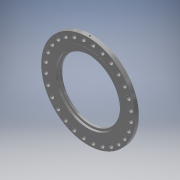
# Autodesk Inventor part: A1-19010-200-01 30in CL300 RFBL flange - thinned
Saved by Autodesk Inventor 2017.3 (Build 213257000, 257)
## iProperties
Created: 2014-07-18
Part Number: A1-19010-200-01 30in CL300 RFBL flange - thinned
Material: Steel, Mild
Document SubType Name: Modeling
Designer: Graeme_Van_Dongen
Density: 7.86 g/cm^3
Appearance: Steel
Mass: 182237 g
Surface Area: 14853.8 cm^2
Volume: 23185.3 cm^3
Description: Ø30" CLASS 300 RFBL FLANGE, A516 Gr.70N, ASME B16.47 Ser.A, 50mm THICK
Author: Graeme_Van_Dongen
Autodesk Inventor part; units mm, degrees
ref_plane "YZ Plane" through (0, 0, 0) normal (1, 0, 0) x (0, 1, 0)
ref_plane "XY Plane" through (0, 0, 0) normal (0, 0, 1) x (1, 0, 0)
sketch "Sketch1" plane through (0, 0, 0) normal (0, 0, 1) x (1, 0, 0)
  circle A0 centre (0, 0) radius 546.1
  dimension "d0" = 1092.2
  constraints: 1 centre point, 1 coincident
  measures "d0" diameter of A0
extrude "Extrusion1" add sketch "Sketch1" along normal blind 48.4125
sketch "Sketch2" plane through (0, 0, 48.4125) normal (0, 0, 1) x (1, 0, 0)
  circle A0 centre (0, 0) radius 428.625
  dimension "d3" = 857.25
  constraints: 1 centre point, 1 coincident
  measures "d3" diameter of A0
extrude "Extrusion2" add sketch "Sketch2" along normal blind 1.5875
sketch "Sketch3" plane through (0, 0, 50) normal (0, 0, 1) x (1, 0, 0)
  circle A0 centre (0, 0) radius 374.65
  dimension "d6" = 749.3
  dimension "d32" = 0
  constraints: 1 centre point, 1 coincident
  measures "d6" diameter of A0
  measures "d32" distance of point (0, 0) A0.centre
extrude "Extrusion3" cut sketch "Sketch3" against normal blind 25.4
sketch "Sketch4" plane through (0, 0, 50) normal (0, 0, 1) x (1, 0, 0)
  circle A0 centre (0, 0) radius 349.25
  circle A1 centre (0, 0) radius 374.65 construction
  dimension "d9" = 698.5
  constraints: 1 centre point, 1 concentric
  measures "d9" diameter of A0
extrude "Extrusion4" cut sketch "Sketch4" against normal through all
sketch "Sketch5" plane through (0, 0, 50) normal (0, 0, 1) x (1, 0, 0)
  line L0 (-495.3407, -55.8115) -> (495.3407, 55.8115)
  line L1 (-495.3407, -55.8115) -> (501.6093, -55.8115) construction
  point P0 (0, 0)
  point P1 (0, 0)
  dimension "d12" = 996.95
  dimension "d13" = 6.429
  constraints: 4 end point, 2 coincident, 1 equal length, 1 horizontal, 1 midpoint
  measures "d12" distance of L0.start L0.end
  measures "d13" angle of L1 L0
hole "Hole1" at (495.3407, 55.8115, 50) direction (0, 0, -1) diameter 47.625 end through all
chamfer "Chamfer3" distance 1.5875 angle 45 2 edges at (495.3407, 79.624, 48.4125) (495.3407, 79.624, 0)
pattern_circular "Circular Pattern1" count 28 over 360 about axis through (0, 0, -10) along (0, 0, 1) of "Hole1", "Chamfer3"
chamfer "Chamfer1" distance 1.5875 angle 45 2 edges at (-546.1, 0, 48.4125) (-546.1, 0, 0)
chamfer "Chamfer2" distance 0.7937 angle 45 1 edges at (-349.25, 0, 24.6)
fillet "Fillet2" radius 0.7937 1 edges at (-374.65, 0, 24.6)
ref_plane "Work Plane1" through (0, 546.1, 0) normal (0, 1, 0) x (-1, 0, 0)
sketch "Sketch6" plane through (0, 546.1, 0) normal (0, 1, 0) x (-1, 0, 0)
  point P0 (0, 0)
  point P1 (0, 24.6062)
  dimension "d36" = 24.6062
  constraints: 1 vertical alignment
  measures "d36" distance of point (0, 0) point (0, 24.606)
hole "Hole2" at (0, 546.1, 24.6062) direction (0, -1, 0) diameter 16.3068 depth 63.5 tip angle 118 thread size "3/4-10 UNC" class "2B" standard "ANSI Unified Screw Threads"
pattern_circular "Circular Pattern2" count 2 over 360 about axis through (0, 0, -10) along (0, 0, 1) of "Hole2"
body "Solid1"
